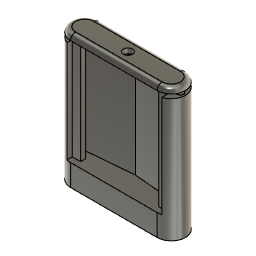
Solar Cell-LED Post (Autodesk Fusion 360 design; units mm, degrees)
Autodesk Fusion 360 part; units mm, degrees
imported_body "Derived Base Feature1" makes body 1 makes body 2 makes body 3 makes body 4 in component "Solar-LED Post"
imported_body "Derived Base Feature2" makes body 5 makes body 6 in component "Solar-LED Post"
move_body "Move1" bodies 5 6 to x (1, 0, 0) y (0, 1, 0) z (0, 0, 1) at (0, 150, 0) in component "Solar-LED Post"
move_body "Move2" bodies 5 6 to x (1, 0, 0) y (0, 1, 0) z (0, 0, 1) at (0, -5, 0) in component "Solar-LED Post"
copy_body "CopyPasteBodies1" bodies 5 makes body 7 in component "Solar-LED Post"
move_body "Move3" bodies 7 to x (1, 0, 0) y (0, 1, 0) z (0, 0, 1) at (-145, 0, 0) in component "Solar-LED Post"
copy_body "CopyPasteBodies2" bodies 5 makes body 8 in component "Solar-LED Post"
move_body "Move4" bodies 8 to x (1, 0, 0) y (0, 1, 0) z (0, 0, 1) at (145, 0, 0) in component "Solar-LED Post"
sketch "Sketch1" plane through (0, 0, 0) normal (0, 1, 0) x (1, 0, 0)
  line L0 (7.5, -69.4031) -> (7.5, -33)
  line L1 (7.5, -33) -> (-7.5, -33)
  line L2 (-7.5, -33) -> (-7.5, -69.4031)
  arc A0 (-7.5, -69.4031) -> (7.5, -69.4031) centre (0, -84.1) ccw
  circle A1 centre (0, -84.1) radius 14
  line L3 (33.1, -112.2) -> (38.1, -112.2)
  line L4 (38.1, -112.2) -> (38.1, -36)
  line L5 (38.1, -36) -> (33.1, -36)
  line L6 (33.1, -36) -> (33.1, -112.2)
  line L7 (-38.1, -112.2) -> (-33.1, -112.2)
  line L8 (-33.1, -112.2) -> (-33.1, -36)
  line L9 (-33.1, -36) -> (-38.1, -36)
  line L10 (-38.1, -36) -> (-38.1, -112.2)
  line L11 (0, -84.1) -> (26.5, -84.1)
  line L12 (26.5, -84.1) -> (26.5, -114.6)
  line L13 (26.5, -114.6) -> (0, -114.6)
  line L14 (0, -114.6) -> (0, -84.1)
  line L15 (0, -84.1) -> (-26.5, -84.1)
  line L16 (-26.5, -84.1) -> (-26.5, -114.6)
  line L17 (-26.5, -114.6) -> (0, -114.6)
  line L18 (0, -114.6) -> (0, -84.1)
  line L19 (0, -84.1) -> (26.5, -84.1)
  line L20 (26.5, -84.1) -> (26.5, -53.6)
  line L21 (26.5, -53.6) -> (0, -53.6)
  line L22 (0, -53.6) -> (0, -84.1)
  line L23 (0, -84.1) -> (-26.5, -84.1)
  line L24 (-26.5, -84.1) -> (-26.5, -53.6)
  line L25 (-26.5, -53.6) -> (0, -53.6)
  line L26 (0, -53.6) -> (0, -84.1)
  line L27 (26.5, -114.6) -> (29.5, -114.6)
  line L28 (29.5, -114.6) -> (29.5, -50.6)
  line L29 (29.5, -50.6) -> (26.5, -50.6)
  line L30 (26.5, -50.6) -> (26.5, -114.6)
  line L31 (-26.5, -114.6) -> (-29.5, -114.6)
  line L32 (-29.5, -114.6) -> (-29.5, -50.6)
  line L33 (-29.5, -50.6) -> (-26.5, -50.6)
  line L34 (-26.5, -50.6) -> (-26.5, -114.6)
  line L35 (-26.5, -50.6) -> (26.5, -50.6)
  line L36 (26.5, -50.6) -> (26.5, -53.6)
  line L37 (26.5, -53.6) -> (-26.5, -53.6)
  line L38 (-26.5, -53.6) -> (-26.5, -50.6)
  dimension "d1" = 26.5
  dimension "d2" = 30.5
  dimension "d3" = 26.5
  dimension "d4" = 30.5
  dimension "d5" = 26.5
  dimension "d6" = 30.5
  dimension "d7" = 3
  dimension "d8" = 64
  dimension "d9" = 3
  dimension "d10" = 64
  constraint horizontal L11
  constraint vertical L12
  constraint horizontal L13
  constraint vertical L14
  constraint coincident A0.centre A1.centre
  constraint horizontal L15
  constraint vertical L16
  constraint horizontal L17
  constraint vertical L18
  constraint horizontal L19
  constraint vertical L20
  constraint horizontal L21
  constraint vertical L22
  constraint horizontal L23
  constraint vertical L24
  constraint horizontal L25
  constraint vertical L26
  constraint horizontal L27
  constraint vertical L28
  constraint horizontal L29
  constraint vertical L30
  constraint horizontal L31
  constraint vertical L32
  constraint horizontal L33
  constraint vertical L34
  constraint horizontal L35
  constraint vertical L36
  constraint horizontal L37
  constraint vertical L38
  measures "d1" distance of A0.centre L11.end
  measures "d2" distance of A0.centre L13.end
  measures "d3" distance of A0.centre L15.end
  measures "d4" distance of A0.centre L13.end
  measures "d5" distance of A0.centre L11.end
  measures "d6" distance of A0.centre L21.end
  measures "d7" distance of L12.end L27.end
  measures "d8" distance of L12.end L29.end
  measures "d9" distance of L16.end L31.end
  measures "d10" distance of L16.end L33.end
extrude "Extrude1" add sketch "Sketch1" along normal blind 15 separate body contours L0 L2 L21 L25 L35 L37 | L0 L21 L30 L35 L36 L37 | L12 L20 L27 L28 L29 L30 L36 | L2 L25 L34 L35 L37 L38 | L16 L24 L31 L32 L33 L34 L38 makes body 9
copy_body "CutPasteBodies3" bodies 9 removing the originals makes body 10 in component "Solar-LED Post"
move_body "Move5" bodies 10 to x (1, 0, 0) y (0, 1, 0) z (0, 0, 1) at (0, 170, 0) in component "Solar-LED Post"
extrude "Extrude1'" add 1 faces at (-29.5, 175, 93.2667) along direction (-1, 0, 0) blind 2 on bodies 10 bodies 10 in component "Solar-LED Post"
extrude "Extrude2" add 1 faces at (29.5, 175, 93.2667) along direction (1, 0, 0) blind 2 on bodies 10 bodies 10 in component "Solar-LED Post"
extrude "Extrude3" cut 1 faces at (-26.5, 175, 94.2667) along direction (-1, 0, 0) blind 2 on bodies 10 bodies 10 in component "Solar-LED Post"
extrude "Extrude4" cut 1 faces at (26.5, 175, 94.2667) along direction (1, 0, 0) blind 2 on bodies 10 bodies 10 in component "Solar-LED Post"
sketch "Sketch2" plane through (0, 0, 53.6) normal (0, 0, 1) x (-1, 0, 0) in component "Solar-LED Post"
  line L0 (28.5, -170) -> (-28.5, -170)
  line L1 (-28.5, -170) -> (-28.5, -185)
  line L2 (-28.5, -185) -> (28.5, -185)
  line L3 (28.5, -185) -> (28.5, -170)
  line L4 (28.5, -185) -> (28.5, -179.5)
  line L5 (28.5, -170) -> (28.5, -175.5)
  line L6 (-28.5, -185) -> (-28.5, -179.5)
  line L7 (-28.5, -170) -> (-28.5, -175.5)
  line L8 (0, -185) -> (0, -182)
  line L9 (0, -182) -> (28.5, -179.5)
  line L10 (0, -182) -> (-28.5, -179.5)
  line L11 (28.5, -170) -> (28.5, -172.5)
  line L12 (-28.5, -170) -> (-28.5, -172.5)
  line L13 (28.5, -175.5) -> (23.5, -175.5)
  line L14 (28.5, -172.5) -> (23.5, -172.5)
  line L15 (23.5, -172.5) -> (23.5, -175.5)
  line L16 (-28.5, -175.5) -> (-23.5, -175.5)
  line L17 (-23.5, -175.5) -> (-23.5, -172.5)
  line L18 (-23.5, -172.5) -> (-28.5, -172.5)
  dimension "d23" = 5.5
  dimension "d24" = 5.5
  dimension "d25" = 5.5
  dimension "d26" = 5.5
  dimension "d27" = 3
  dimension "d30" = 2.5
  dimension "d31" = 2.5
  dimension "d32" = 5
  dimension "d33" = 5
  constraint coincident L2.end L3.start
  constraint coincident L3 L4.end
  constraint coincident L0.start L3.end
  constraint coincident L3 L5.end
  constraint coincident L1.end L2.start
  constraint coincident L1 L6.end
  constraint coincident L0.end L1.start
  constraint perpendicular L0 L7
  constraint midpoint L2 L8.start
  constraint perpendicular L2 L8
  constraint perpendicular L0 L11
  constraint perpendicular L0 L12
  constraint perpendicular L5 L13
  constraint perpendicular L5 L14
  constraint perpendicular L13 L15
  constraint perpendicular L7 L16
  constraint perpendicular L16 L17
  constraint perpendicular L12 L18
  measures "d23" distance of L2.end L4.end
  measures "d24" distance of L0.start L5.end
  measures "d25" distance of L1.end L6.end
  measures "d26" distance of L0.end L7.end
  measures "d27" distance of L8.start L8.end
  measures "d30" distance of L0.start L11.end
  measures "d31" distance of L0.end L12.end
  measures "d32" distance of L5.end L13.end
  measures "d33" distance of L7.end L16.end
extrude "Extrude5" add sketch "Sketch2" along normal up to surface (61 mm away) contours L2 L3 L4 L8 L9 | L1 L2 L6 L8 L10 bodies 10 in component "Solar-LED Post"
extrude "Extrude6" add sketch "Sketch2" along normal up to surface (61 mm away) contours L3 L5 L13 L14 L15 | L1 L7 L16 L17 L18 bodies 10 in component "Solar-LED Post"
extrude "Extrude7" add 1 faces at (31.5, 175, 93.2667) along direction (1, 0, 0) blind 3 on bodies 10 bodies 10 in component "Solar-LED Post"
extrude "Extrude8" add 1 faces at (-31.5, 175, 93.2667) along direction (-1, 0, 0) blind 3 on bodies 10 bodies 10 in component "Solar-LED Post"
sketch "Sketch3" plane through (0, 0, 114.6) normal (0, 0, 1) x (-1, 0, 0) in component "Solar-LED Post"
  line L0 (28.5, -170) -> (28.5, -172.5)
  line L1 (28.5, -172.5) -> (23.5, -172.5)
  line L2 (23.5, -172.5) -> (23.5, -175.5)
  line L3 (23.5, -175.5) -> (28.5, -175.5)
  line L4 (28.5, -175.5) -> (28.5, -179.5)
  line L5 (28.5, -179.5) -> (0, -182)
  line L6 (0, -182) -> (-28.5, -179.5)
  line L7 (-28.5, -179.5) -> (-28.5, -175.5)
  line L8 (-28.5, -175.5) -> (-23.5, -175.5)
  line L9 (-23.5, -175.5) -> (-23.5, -172.5)
  line L10 (-23.5, -172.5) -> (-28.5, -172.5)
  line L11 (-28.5, -172.5) -> (-28.5, -170)
  line L12 (-28.5, -170) -> (-34.5, -170)
  line L13 (-34.5, -170) -> (-34.5, -185)
  line L14 (-34.5, -185) -> (34.5, -185)
  line L15 (34.5, -185) -> (34.5, -170)
  line L16 (34.5, -170) -> (28.5, -170)
  line L17 (34.5, -185) -> (28.5, -179.5) construction
  line L18 (34.5, -170) -> (28.5, -175.5) construction
  line L19 (-28.5, -179.5) -> (-34.5, -185) construction
  line L20 (-28.5, -175.5) -> (-34.5, -170) construction
  circle A0 centre (-31.5, -182.25) radius 2
  circle A1 centre (-31.5, -172.75) radius 2
  circle A2 centre (31.5, -182.25) radius 2
  circle A3 centre (31.5, -172.75) radius 2
  dimension "d40" = 4
  dimension "d41" = 4
  dimension "d42" = 4
  dimension "d43" = 4
  constraint coincident L14.end L15.start
  constraint coincident L4.end L5.start
  constraint coincident L15.end L16.start
  constraint coincident L3.end L4.start
  constraint coincident L6.end L7.start
  constraint coincident L13.end L14.start
  constraint coincident L7.end L8.start
  constraint coincident L12.end L13.start
  constraint midpoint L19 A0.centre
  constraint midpoint L20 A1.centre
  constraint midpoint L17 A2.centre
  constraint midpoint L18 A3.centre
  measures "d40" diameter of A0
  measures "d41" diameter of A1
  measures "d42" diameter of A2
  measures "d43" diameter of A3
extrude "Extrude9" add 1 faces at (-32.5, 170, 72.9333) along direction (0, -1, 0) blind 1 on bodies 10 bodies 10 in component "Solar-LED Post"
extrude "Extrude10" add 1 faces at (-11.5, 185, 71.9333) along direction (0, 1, 0) blind 1 on bodies 10 bodies 10 in component "Solar-LED Post"
extrude "Extrude11" cut sketch "Sketch3" against normal blind 3 contours A0 | A1 | A2 | A3 bodies 10 in component "Solar-LED Post"
sketch "Sketch4" plane through (0, 0, 114.6) normal (0, 0, 1) x (-1, 0, 0) in component "Solar-LED Post"
  circle A0 centre (31.5, -172.75) radius 2
  circle A1 centre (-31.5, -182.25) radius 2
  circle A2 centre (31.5, -182.25) radius 2
  circle A3 centre (-31.5, -172.75) radius 2
  line L0 (28.5, -169) -> (28.5, -172.5)
  line L1 (28.5, -172.5) -> (23.5, -172.5)
  line L2 (23.5, -172.5) -> (23.5, -175.5)
  line L3 (23.5, -175.5) -> (28.5, -175.5)
  line L4 (28.5, -175.5) -> (28.5, -179.5)
  line L5 (28.5, -179.5) -> (0, -182)
  line L6 (0, -182) -> (-28.5, -179.5)
  line L7 (-28.5, -179.5) -> (-28.5, -175.5)
  line L8 (-28.5, -175.5) -> (-23.5, -175.5)
  line L9 (-23.5, -175.5) -> (-23.5, -172.5)
  line L10 (-23.5, -172.5) -> (-28.5, -172.5)
  line L11 (-28.5, -172.5) -> (-28.5, -169)
  line L12 (-28.5, -169) -> (-34.5, -169)
  line L13 (-34.5, -169) -> (-34.5, -186)
  line L14 (-34.5, -186) -> (34.5, -186)
  line L15 (34.5, -186) -> (34.5, -169)
  line L16 (34.5, -169) -> (28.5, -169)
  line L17 (34.5, -186) -> (-34.5, -186)
  line L18 (-34.5, -186) -> (-34.5, -169)
  line L19 (-34.5, -169) -> (34.5, -169)
  line L20 (34.5, -169) -> (34.5, -186)
  constraint horizontal L17
  constraint vertical L18
  constraint horizontal L19
  constraint vertical L20
  constraint coincident L12.end L13.start
  constraint coincident L14.end L15.start
extrude "Extrude12" add sketch "Sketch4" along normal blind 2.5 separate body contours A0 | A1 | A2 | A3 makes body 11 at (29.5618, 172.2565, 116.2667) makes body 12 at (-29.5618, 181.7565, 116.2667) makes body 13 at (33.0321, 183.5356, 116.2667) makes body 14 at (-29.5618, 172.2565, 116.2667) in component "Solar-LED Post"
sketch "Sketch5" plane through (0, 0, 117.1) normal (0, 0, 1) x (-1, 0, 0) in component "Solar-LED Post"
  circle A0 centre (31.5, -182.25) radius 2
  circle A1 centre (31.5, -172.75) radius 2
  circle A2 centre (-31.5, -182.25) radius 2
  circle A3 centre (31.5, -182.25) radius 2
  circle A4 centre (-31.5, -172.75) radius 2
  line L0 (28.5, -169) -> (28.5, -172.5)
  line L1 (28.5, -172.5) -> (23.5, -172.5)
  line L2 (23.5, -172.5) -> (23.5, -175.5)
  line L3 (23.5, -175.5) -> (28.5, -175.5)
  line L4 (28.5, -175.5) -> (28.5, -179.5)
  line L5 (28.5, -179.5) -> (0, -182)
  line L6 (0, -182) -> (-28.5, -179.5)
  line L7 (-28.5, -179.5) -> (-28.5, -175.5)
  line L8 (-28.5, -175.5) -> (-23.5, -175.5)
  line L9 (-23.5, -175.5) -> (-23.5, -172.5)
  line L10 (-23.5, -172.5) -> (-28.5, -172.5)
  line L11 (-28.5, -172.5) -> (-28.5, -169)
  line L12 (-28.5, -169) -> (-34.5, -169)
  line L13 (-34.5, -169) -> (-34.5, -186)
  line L14 (-34.5, -186) -> (34.5, -186)
  line L15 (34.5, -186) -> (34.5, -169)
  line L16 (34.5, -169) -> (28.5, -169)
  line L17 (34.5, -186) -> (-34.5, -186)
  line L18 (-34.5, -186) -> (-34.5, -169)
  line L19 (-34.5, -169) -> (34.5, -169)
  line L20 (34.5, -169) -> (34.5, -186)
  constraint horizontal L17
  constraint vertical L18
  constraint horizontal L19
  constraint vertical L20
  constraint coincident L12.end L13.start
  constraint coincident L14.end L15.start
extrude "Extrude13" add sketch "Sketch5" along normal blind 3 contours A0 A3 | A1 | A2 | A4 | L0 L1 L2 L3 L4 L5 L6 L7 L8 L9 L10 L11 L12 L13 L14 L15 L16 L17 L18 L19 L20 | L0 L1 L2 L3 L4 L5 L6 L7 L8 L9 L10 L11 L19 bodies 11 12 13 14 in component "Solar-LED Post"
sketch "Sketch6" plane through (0, 0, 120.1) normal (0, 0, 1) x (-1, 0, 0) in component "Solar-LED Post"
  line L0 (34.5, -169) -> (-34.5, -169)
  line L1 (-34.5, -169) -> (-34.5, -186)
  line L2 (-34.5, -186) -> (34.5, -186)
  line L3 (34.5, -186) -> (34.5, -169)
  circle A0 centre (0, -177.5) radius 3
  dimension "d54" = 6
  measures "d54" diameter of A0
extrude "Extrude14" cut sketch "Sketch6" against normal up to surface (3 mm away) contours A0 bodies 11 in component "Solar-LED Post"
extrude "Extrude15" add 1 faces at (11.5, 174.6667, 50.6) along direction (0, 0, -1) blind 10 on bodies 10 bodies 10 in component "Solar-LED Post"
sketch "Sketch7" plane through (0, 0, 40.6) normal (0, 0, -1) x (1, 0, 0) in component "Solar-LED Post"
  line L0 (-34.5, -169) -> (-34.5, -186)
  line L1 (-34.5, -186) -> (34.5, -186)
  line L2 (34.5, -186) -> (34.5, -169)
  line L3 (34.5, -169) -> (-34.5, -169)
  circle A0 centre (0, -177.5) radius 5.25
  dimension "d59" = 10.5
  measures "d59" diameter of A0
extrude "Extrude16" cut sketch "Sketch7" against normal blind 10 contours A0 bodies 10 in component "Solar-LED Post"
sketch "Sketch2 (2)" plane through (0, 0, 114.6) normal (0, 0, -1) x (1, 0, 0)
  circle A0 centre (31.5, -172.75) radius 2
  circle A1 centre (31.5, -172.75) radius 1.5
  circle A2 centre (31.5, -182.25) radius 2
  circle A3 centre (-31.5, -182.25) radius 2
  circle A4 centre (-31.5, -172.75) radius 2
  circle A5 centre (-31.5, -172.75) radius 1.5
  circle A6 centre (-31.5, -182.25) radius 1.5
  circle A7 centre (31.5, -182.25) radius 1.5
  dimension "d62" = 3
  dimension "d63" = 3
  dimension "d64" = 3
  dimension "d65" = 3
  constraint concentric A0 A1
  constraint concentric A4 A5
  constraint concentric A3 A6
  constraint concentric A2 A7
  measures "d62" diameter of A1
  measures "d63" diameter of A5
  measures "d64" diameter of A6
  measures "d65" diameter of A7
extrude "Extrude17" cut sketch "Sketch2 (2)" against normal up to surface (2.5 mm away) bodies 11 in component "Solar-LED Post"
sketch "Sketch3 (2)" plane through (0, 0, 117.1) normal (0, 0, -1) x (1, 0, 0)
  circle A0 centre (31.5, -172.75) radius 1.5
  circle A1 centre (-31.5, -172.75) radius 1.5
  circle A2 centre (31.5, -182.25) radius 1.5
  circle A3 centre (-31.5, -182.25) radius 1.5
  circle A4 centre (0, -177.5) radius 3
  line L0 (34.5, -169) -> (-34.5, -169)
  line L1 (-34.5, -169) -> (-34.5, -186)
  line L2 (-34.5, -186) -> (34.5, -186)
  line L3 (34.5, -186) -> (34.5, -169)
  circle A5 centre (0, -177.5) radius 2.75
  dimension "d68" = 5.5
  constraint concentric A4 A5
  measures "d68" diameter of A5
extrude "Extrude18" add sketch "Sketch3 (2)" against normal up to surface (3 mm away) contours A4 bodies 11 in component "Solar-LED Post"
sketch "Sketch8" plane through (0, 0, 117.1) normal (0, 0, -1) x (1, 0, 0) in component "Solar-LED Post"
  circle A0 centre (0, -177.5) radius 2.75
  circle A1 centre (31.5, -172.75) radius 1.5
  circle A2 centre (-31.5, -172.75) radius 1.5
  circle A3 centre (31.5, -182.25) radius 1.5
  circle A4 centre (-31.5, -182.25) radius 1.5
  line L0 (34.5, -169) -> (-34.5, -169)
  line L1 (-34.5, -169) -> (-34.5, -186)
  line L2 (-34.5, -186) -> (34.5, -186)
  line L3 (34.5, -186) -> (34.5, -169)
  circle A5 centre (31.5, -172.75) radius 1.75
  circle A6 centre (31.5, -182.25) radius 1.75
  circle A7 centre (-31.5, -182.25) radius 1.75
  circle A8 centre (-31.5, -172.75) radius 1.75
  dimension "d71" = 3.5
  dimension "d72" = 3.5
  dimension "d73" = 3.5
  dimension "d74" = 3.5
  constraint concentric A1 A5
  constraint concentric A3 A6
  constraint concentric A4 A7
  constraint concentric A2 A8
  measures "d71" diameter of A5
  measures "d72" diameter of A6
  measures "d73" diameter of A7
  measures "d74" diameter of A8
extrude "Extrude19" add sketch "Sketch8" along normal up to surface (2.5 mm away) contours A5 | A6 | A7 | A8 bodies 11 in component "Solar-LED Post"
extrude "Extrude20" add 4 faces at (30.9453, 181.5073, 111.6) (31.9378, 173.5671, 111.6) (-30.8408, 181.2437, 111.6) (-31.0843, 171.8358, 111.6) along direction (0, 0, 1) up to surface end surface through (34.5, 185, 114.6) normal (0, 0, 1) offset 0 on bodies 10 bodies 10 in component "Solar-LED Post"
fillet "Fillet1" radius 8.5 2 edges at (-34.5, 169, 77.6) (-34.5, 186, 77.6) on bodies 10 in component "Solar-LED Post"
fillet "Fillet1" radius 8.5 2 edges at (34.5, 169, 77.6) (34.5, 186, 77.6) on bodies 10 in component "Solar-LED Post"
extrude "Extrude21" cut 4 faces at (-32.199, 182.7826, 114.6) (-30.8128, 172.3532, 114.6) (32.4324, 173.1846, 114.6) (32.1872, 181.8532, 114.6) along direction (0, 0, -1) up to surface end surface through (0, 0, 117.1) normal (0, 0, -1) offset 0 on bodies 11 bodies 11 in component "Solar-LED Post"
fillet "Fillet2" radius 8.5 4 edges at (34.5, 186, 118.6) (34.5, 169, 118.6) (-34.5, 169, 118.6) (-34.5, 186, 118.6) on bodies 11 in component "Solar-LED Post"
sketch "Sketch9" plane through (0, 0, 114.6) normal (0, 0, 1) x (-1, 0, 0) in component "Solar-LED Post"
  arc A0 (-28.5, -169.376) -> (-26, -186) centre (-26, -177.5) ccw
  line L0 (-26, -186) -> (26, -186)
  arc A1 (26, -186) -> (28.5, -169.376) centre (26, -177.5) ccw
  line L1 (28.5, -169.376) -> (28.5, -172.5)
  line L2 (28.5, -172.5) -> (23.5, -172.5)
  line L3 (23.5, -172.5) -> (23.5, -175.5)
  line L4 (23.5, -175.5) -> (28.5, -175.5)
  line L5 (28.5, -175.5) -> (28.5, -179.5)
  line L6 (28.5, -179.5) -> (0, -182)
  line L7 (0, -182) -> (-28.5, -179.5)
  line L8 (-28.5, -179.5) -> (-28.5, -175.5)
  line L9 (-28.5, -175.5) -> (-23.5, -175.5)
  line L10 (-23.5, -175.5) -> (-23.5, -172.5)
  line L11 (-23.5, -172.5) -> (-28.5, -172.5)
  line L12 (-28.5, -172.5) -> (-28.5, -169.376)
  arc A2 (-26, -169) -> (-28.5, -169.376) centre (-26, -177.5) ccw construction
  line L13 (-28.5, -169.376) -> (-28.5, -172.5) construction
  line L14 (-28.5, -172.5) -> (-23.5, -172.5) construction
  line L15 (-23.5, -172.5) -> (-23.5, -175.5) construction
  line L16 (-23.5, -175.5) -> (-28.5, -175.5) construction
  line L17 (-28.5, -175.5) -> (-28.5, -179.5) construction
  line L18 (-28.5, -179.5) -> (0, -182) construction
  line L19 (0, -182) -> (28.5, -179.5) construction
  line L20 (28.5, -179.5) -> (28.5, -175.5) construction
  line L21 (28.5, -175.5) -> (23.5, -175.5) construction
  line L22 (23.5, -175.5) -> (23.5, -172.5) construction
  line L23 (23.5, -172.5) -> (28.5, -172.5) construction
  line L24 (28.5, -172.5) -> (28.5, -169.376) construction
  arc A3 (28.5, -169.376) -> (26, -169) centre (26, -177.5) ccw construction
  line L25 (26, -169) -> (-26, -169) construction
  line L26 (0, -186) -> (0, -169) construction
  line L27 (0, -186) -> (0, -177.5) construction
  line L28 (0, -177.5) -> (34.5, -177.5) construction
  line L29 (34.5, -177.5) -> (31.5, -177.5) construction
  circle A4 centre (31.5, -177.5) radius 2
  line L30 (0, -177.5) -> (-34.5, -177.5) construction
  line L31 (-34.5, -177.5) -> (-31.5, -177.5) construction
  circle A5 centre (-31.5, -177.5) radius 2
  dimension "d87" = 8.5
  dimension "d88" = 3
  dimension "d89" = 4
  dimension "d90" = 3
  dimension "d91" = 4
  constraint midpoint L0 L26.start
  constraint midpoint L25 L26.end
  constraint midpoint L26 L27.end
  constraint coincident A1 L28.end
  constraint perpendicular L5 L28
  constraint coincident L28 L29.end
  constraint coincident L29.end A4.centre
  constraint coincident A0 L30.end
  constraint perpendicular L17 L30
  constraint coincident L30 L31.end
  constraint coincident L31.end A5.centre
  measures "d87" distance of L26.start L27.end
  measures "d88" distance of L28.end L29.end
  measures "d89" diameter of A4
  measures "d90" distance of L30.end L31.end
  measures "d91" diameter of A5
extrude "Extrude22" cut sketch "Sketch9" against normal blind 3 contours A4 | A5 bodies 10 in component "Solar-LED Post"
sketch "Sketch10" plane through (0, 0, 117.1) normal (0, 0, -1) x (1, 0, 0) in component "Solar-LED Post"
  arc A0 (-26, -169) -> (-26, -186) centre (-26, -177.5) ccw
  line L0 (-26, -186) -> (26, -186)
  arc A1 (26, -186) -> (26, -169) centre (26, -177.5) ccw
  line L1 (26, -169) -> (-26, -169)
  circle A2 centre (0, -177.5) radius 2.75
  circle A3 centre (-31.5, -177.5) radius 2
  circle A4 centre (31.5, -177.5) radius 2
  circle A5 centre (-31.5, -177.5) radius 1.75
  circle A6 centre (31.5, -177.5) radius 1.75
  dimension "d94" = 3.5
  dimension "d95" = 3.5
  constraint concentric A3 A5
  constraint concentric A4 A6
  measures "d94" diameter of A5
  measures "d95" diameter of A6
extrude "Extrude23" add sketch "Sketch10" along normal blind 2.5 contours A5 | A6 bodies 11 in component "Solar-LED Post"
fillet "Fillet3" radius 3 4 edges at (0, 169, 120.1) (-34.5, 177.5, 120.1) (0, 186, 120.1) (34.5, 177.5, 120.1) on bodies 11 in component "Solar-LED Post"
component "Solar-LED Post" placed x (1, 0, 0) y (0, 1, 0) z (0, 0, 1) at (0, 0, 0)
hidden bodies 1 2 3 4 5 6 7 8
named bodies: "Optical Breadboard", "Mirror Slot Post", "Body3", "Body5", "Optical Breadboard (1)", "Quarter Circle Slidetrack Post", "Optical Breadboard (1) (1)", "Optical Breadboard (1) (2)"
